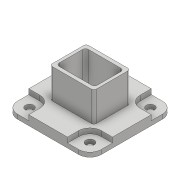
# Autodesk Inventor part: RJ45Panel
Saved by Autodesk Inventor 2017 (Build 210142000, 142)
## iProperties
Created: 2017-11-20
Part Number: RJ45Panel
Material: Generic
Document SubType Name: Modeling
Designer: Kathryn Rosie
Density: 1 g/cm^3
Appearance: Default
Author: Kathryn Rosie
Autodesk Inventor part; units mm, degrees
ref_plane "YZ Plane" through (0, 0, 0) normal (1, 0, 0) x (0, 1, 0)
ref_plane "XZ Plane" through (0, 0, 0) normal (0, 1, 0) x (-1, 0, 0)
ref_plane "XY Plane" through (0, 0, 0) normal (0, 0, 1) x (1, 0, 0)
sketch "Sketch1" plane through (0, 0, 0) normal (0, 0, 1) x (1, 0, 0)
  line L0 (-12.55, -17.15) -> (12.55, -17.15)
  line L1 (17.15, -12.55) -> (17.15, 12.55)
  line L2 (12.55, 17.15) -> (-12.55, 17.15)
  line L3 (-17.15, 12.55) -> (-17.15, -12.55)
  line L4 (-17.15, -17.15) -> (17.15, 17.15) construction
  line L5 (17.15, -17.15) -> (-17.15, 17.15) construction
  circle A0 centre (0, 0) radius 17.5 construction
  circle A1 centre (-12.3744, 12.3744) radius 1.7
  circle A2 centre (-12.3744, -12.3744) radius 1.7
  circle A3 centre (12.3744, -12.3744) radius 1.7
  circle A4 centre (12.3744, 12.3744) radius 1.7
  line L6 (-12.3744, 12.3744) -> (-12.3744, 17.15) construction
  line L7 (-12.3744, 12.3744) -> (-7.5987, 12.3744) construction
  arc A5 (-12.55, 17.15) -> (-17.15, 12.55) centre (-12.55, 12.55) ccw
  arc A6 (17.15, 12.55) -> (12.55, 17.15) centre (12.55, 12.55) ccw
  arc A7 (12.55, -17.15) -> (17.15, -12.55) centre (12.55, -12.55) ccw
  arc A8 (-17.15, -12.55) -> (-12.55, -17.15) centre (-12.55, -12.55) ccw
  line L8 (-8.025, -7.45) -> (8.025, -7.45)
  line L9 (9.025, -6.45) -> (9.025, 6.45)
  line L10 (8.025, 7.45) -> (-8.025, 7.45)
  line L11 (-9.025, 6.45) -> (-9.025, -6.45)
  line L12 (-9.025, -7.45) -> (9.025, 7.45) construction
  line L13 (9.025, -7.45) -> (-9.025, 7.45) construction
  arc A9 (-8.025, 7.45) -> (-9.025, 6.45) centre (-8.025, 6.45) ccw
  arc A10 (9.025, 6.45) -> (8.025, 7.45) centre (8.025, 6.45) ccw
  arc A11 (8.025, -7.45) -> (9.025, -6.45) centre (8.025, -6.45) ccw
  arc A12 (-9.025, -6.45) -> (-8.025, -7.45) centre (-8.025, -6.45) ccw
  dimension "d0" = 34.3
  dimension "d1" = 34.3
  dimension "d2" = 35
  dimension "d3" = 3.4
  dimension "d4" = 3.4
  dimension "d5" = 3.4
  dimension "d6" = 3.4
  dimension "d7" = 90
  dimension "d8" = 4.6
  dimension "d9" = 18.05
  dimension "d10" = 14.9
  dimension "d11" = 1
  constraints: 28 end point, 21 point on line, 20 point on circle, 16 tangent, 13 centre point, 6 equal radius, 4 midpoint, 4 parallel, 3 horizontal, 3 perpendicular, 1 coincident
  measures "d0" distance of L5.end L4.end
  measures "d1" distance of L4.end L5.start
  measures "d2" diameter of A0
  measures "d3" diameter of A1
  measures "d4" diameter of A2
  measures "d5" diameter of A3
  measures "d6" diameter of A4
  measures "d7" angle of L7 L6
  measures "d8" radius of A5
  measures "d9" distance of L13.end L12.end
  measures "d10" distance of L12.end L13.start
  measures "d11" radius of A9
extrude "Extrusion1" add sketch "Sketch1" along normal blind 3.9
sketch "Sketch2" plane through (0, 0, 3.9) normal (0, 0, 1) x (1, 0, 0)
  arc A0 (9.025, 6.45) -> (8.025, 7.45) centre (8.025, 6.45) ccw projected
  line L0 (9.025, 6.45) -> (9.025, -6.45) projected
  arc A1 (8.025, -7.45) -> (9.025, -6.45) centre (8.025, -6.45) ccw projected
  line L1 (8.025, -7.45) -> (-8.025, -7.45) projected
  arc A2 (-9.025, -6.45) -> (-8.025, -7.45) centre (-8.025, -6.45) ccw projected
  line L2 (-9.025, -6.45) -> (-9.025, 6.45) projected
  arc A3 (-8.025, 7.45) -> (-9.025, 6.45) centre (-8.025, 6.45) ccw projected
  line L3 (-8.025, 7.45) -> (8.025, 7.45) projected
  circle A4 centre (12.3744, 12.3744) radius 1.7 projected
  circle A5 centre (12.3744, -12.3744) radius 1.7 projected
  circle A6 centre (-12.3744, -12.3744) radius 1.7 projected
  circle A7 centre (-12.3744, 12.3744) radius 1.7 projected
  line L4 (-17.15, 12.55) -> (-17.15, -12.55) projected
  arc A8 (-17.15, -12.55) -> (-12.55, -17.15) centre (-12.55, -12.55) ccw projected
  line L5 (-12.55, -17.15) -> (12.55, -17.15) projected
  arc A9 (12.55, -17.15) -> (17.15, -12.55) centre (12.55, -12.55) ccw projected
  line L6 (17.15, -12.55) -> (17.15, 12.55) projected
  arc A10 (17.15, 12.55) -> (12.55, 17.15) centre (12.55, 12.55) ccw projected
  line L7 (12.55, 17.15) -> (-12.55, 17.15) projected
  arc A11 (-12.55, 17.15) -> (-17.15, 12.55) centre (-12.55, 12.55) ccw projected
  line L8 (12.55, 7.95) -> (17.15, 7.95)
  line L9 (17.15, 7.95) -> (17.15, 12.55)
  line L10 (12.55, 17.15) -> (7.95, 17.15)
  line L11 (7.95, 17.15) -> (7.95, 12.55)
  line L12 (7.95, 7.95) -> (17.15, 17.15) construction
  line L13 (17.15, 7.95) -> (7.95, 17.15) construction
  arc A12 (7.95, 12.55) -> (12.55, 7.95) centre (12.55, 12.55) ccw
  arc A13 (17.15, 12.55) -> (12.55, 17.15) centre (12.55, 12.55) ccw
  line L14 (-12.55, 7.95) -> (-17.15, 7.95)
  line L15 (-17.15, 7.95) -> (-17.15, 12.55)
  line L16 (-12.55, 17.15) -> (-7.95, 17.15)
  line L17 (-7.95, 17.15) -> (-7.95, 12.55)
  line L18 (-7.95, 7.95) -> (-17.15, 17.15) construction
  line L19 (-17.15, 7.95) -> (-7.95, 17.15) construction
  line L20 (-12.55, -7.95) -> (-17.15, -7.95)
  line L21 (-17.15, -7.95) -> (-17.15, -12.55)
  line L22 (-12.55, -17.15) -> (-7.95, -17.15)
  line L23 (-7.95, -17.15) -> (-7.95, -12.55)
  line L24 (-7.95, -7.95) -> (-17.15, -17.15) construction
  line L25 (-17.15, -7.95) -> (-7.95, -17.15) construction
  line L26 (12.55, -7.95) -> (17.15, -7.95)
  line L27 (17.15, -7.95) -> (17.15, -12.55)
  line L28 (12.55, -17.15) -> (7.95, -17.15)
  line L29 (7.95, -17.15) -> (7.95, -12.55)
  line L30 (7.95, -7.95) -> (17.15, -17.15) construction
  line L31 (17.15, -7.95) -> (7.95, -17.15) construction
  arc A14 (12.55, -7.95) -> (7.95, -12.55) centre (12.55, -12.55) ccw
  arc A15 (12.55, -17.15) -> (17.15, -12.55) centre (12.55, -12.55) ccw
  arc A16 (-7.95, -12.55) -> (-12.55, -7.95) centre (-12.55, -12.55) ccw
  arc A17 (-17.15, -12.55) -> (-12.55, -17.15) centre (-12.55, -12.55) ccw
  arc A18 (-12.55, 17.15) -> (-17.15, 12.55) centre (-12.55, 12.55) ccw
  arc A19 (-12.55, 7.95) -> (-7.95, 12.55) centre (-12.55, 12.55) ccw
  constraints: 48 end point, 16 point on circle, 8 centre point, 8 midpoint, 8 parallel, 8 point on line, 4 coincident, 4 horizontal, 4 perpendicular
extrude "Extrusion2" cut sketch "Sketch2" against normal blind 2.1 contours A11 L7 L17 A19 L14 L4 | L20 A16 L23 L5 A8 L4 | L7 A10 L6 L8 A12 L11 | L29 A14 L26 L6 A9 L5
sketch "Sketch3" plane through (0, 0, 3.9) normal (0, 0, 1) x (1, 0, 0)
  line L0 (-6.597, -6.009) -> (6.597, -6.009)
  line L1 (7.85, -4.756) -> (7.85, 4.756)
  line L2 (6.597, 6.009) -> (-6.597, 6.009)
  line L3 (-7.85, 4.756) -> (-7.85, -4.756)
  line L4 (-7.85, -6.009) -> (7.85, 6.009) construction
  line L5 (7.85, -6.009) -> (-7.85, 6.009) construction
  arc A0 (-6.597, 6.009) -> (-7.85, 4.756) centre (-6.597, 4.756) ccw
  arc A1 (7.85, 4.756) -> (6.597, 6.009) centre (6.597, 4.756) ccw
  arc A2 (6.597, -6.009) -> (7.85, -4.756) centre (6.597, -4.756) ccw
  arc A3 (-7.85, -4.756) -> (-6.597, -6.009) centre (-6.597, -4.756) ccw
  line L6 (-8.025, 7.45) -> (8.025, 7.45) projected
  arc A4 (-8.025, 7.45) -> (-9.025, 6.45) centre (-8.025, 6.45) ccw projected
  line L7 (-9.025, -6.45) -> (-9.025, 6.45) projected
  arc A5 (-9.025, -6.45) -> (-8.025, -7.45) centre (-8.025, -6.45) ccw projected
  line L8 (8.025, -7.45) -> (-8.025, -7.45) projected
  arc A6 (8.025, -7.45) -> (9.025, -6.45) centre (8.025, -6.45) ccw projected
  line L9 (9.025, 6.45) -> (9.025, -6.45) projected
  arc A7 (9.025, 6.45) -> (8.025, 7.45) centre (8.025, 6.45) ccw projected
  point P0 (0, 0)
  dimension "d25" = 15.7
  dimension "d26" = 12.018
  dimension "d27" = 1.253
  constraints: 12 end point, 8 point on circle, 8 point on line, 8 tangent, 4 centre point, 3 equal radius, 2 midpoint, 2 parallel, 1 horizontal, 1 perpendicular
  measures "d25" distance of L5.end L4.end
  measures "d26" distance of L4.end L5.start
  measures "d27" radius of A0
extrude "Extrusion3" add sketch "Sketch3" along normal blind 12.2
body "Solid1"
